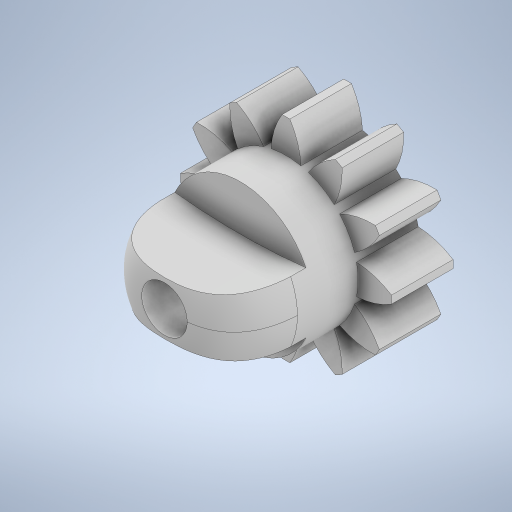
# Autodesk Inventor part: 가스벨브 기어
Saved by Autodesk Inventor 2023.1 (Build 271208000, 208)
## iProperties
Created: 2022-08-14
Part Number: 가스벨브 기어
Material: 일반
Document SubType Name: Modeling
Designer: fly01
Density: 1 g/cm^3
Appearance: 기본값
Author: fly01
Autodesk Inventor part; units mm, degrees
ref_plane "YZ Plane" through (0, 0, 0) normal (1, 0, 0) x (0, 1, 0)
ref_plane "XZ Plane" through (0, 0, 0) normal (0, 1, 0) x (-1, 0, 0)
ref_plane "XY Plane" through (0, 0, 0) normal (0, 0, 1) x (1, 0, 0)
sketch "스케치1" plane through (0, 0, 0) normal (0, 0, 1) x (1, 0, 0)
  circle A0 centre (0, 0) radius 12 construction
  circle A1 centre (0, 0) radius 14
  circle A2 centre (0, 0) radius 9.5
  line L0 (0, 16.0877) -> (0, 8.5475) construction
  line L1 (-0.57, 16.0877) -> (-0.57, 8.5475) construction
  line L2 (-1.57, 16.0877) -> (-1.57, 8.5475) construction
  line L3 (-2.07, 16.0877) -> (-2.07, 8.5475) construction
  arc A3 (-0.57, 13.9884) -> (-2.07, 9.2717) centre (7.6252, 8.7853) ccw
  arc A4 (2.07, 9.2717) -> (0.57, 13.9884) centre (-7.6252, 8.7853) ccw
  circle A5 centre (0, 0) radius 3.75
  line L4 (-3.75, 2.45) -> (3.75, 2.45)
  line L5 (3.75, 2.45) -> (3.75, -2.45)
  line L6 (3.75, -2.45) -> (-3.75, -2.45)
  line L7 (-3.75, -2.45) -> (-3.75, 2.45)
  line L8 (-3.75, 2.45) -> (3.75, -2.45) construction
  line L9 (3.75, 2.45) -> (-3.75, -2.45) construction
  point P0 (2.839, 2.45)
  point P1 (2.839, -2.45)
  point P2 (-2.839, -2.45)
  point P3 (-2.839, 2.45)
  point P4 (2.07, 9.2717)
  point P5 (0.57, 13.9884)
  dimension "d1" = 28
  dimension "d2" = 19
  dimension "d0" = 24
  dimension "d3" = 1.57
  dimension "d4" = 1
  dimension "d5" = 0.5
  dimension "d6" = 7.5
  dimension "d7" = 4.9
  constraints: 20 end point, 5 parallel, 4 centre point, 4 coincident, 4 point on circle, 3 symmetric about line, 2 midpoint, 2 point on line, 1 horizontal, 1 perpendicular, 1 vertical, 1 vertical alignment, 7 other
  measures "d0" diameter of A0
  measures "d3" distance between parallel lines of L0 L2
  measures "d4" distance between parallel lines of L2 L1
  measures "d5" distance between parallel lines of L3 L2
  measures "d6" diameter of A5
  measures "d7" distance of L4.end L5.end
extrude "돌출1" add sketch "스케치1" along normal blind 8.1 contours A2 | A5 L6 L4 | L5 L6 A5 | A5 L4 L5 | L4 A5 | A5 L6 | A5 L7 L4 | L6 L7 A5
extrude "돌출2" add sketch "스케치1" along normal blind 8.1 contours A4 A2 A3 A1 picked at (0.4463, 11.4518)
extrude "돌출3" cut sketch "스케치1" along normal blind 4.1 contours A5 L6 L4
sketch "스케치2" plane through (0, 0, 8.1) normal (0, 0, 1) x (1, 0, 0)
  circle A0 centre (0, 0) radius 1.75
  dimension "d14" = 3.5
  constraints: 1 centre point, 1 coincident
  measures "d14" diameter of A0
extrude "돌출4" cut sketch "스케치2" against normal through all
sketch "스케치4" plane through (0, 0, 8.1) normal (0, 0, 1) x (1, 0, 0)
  circle A0 centre (0, 0) radius 1.75 projected
  arc A1 (-2.07, 9.2717) -> (2.07, 9.2717) centre (0, 0) ccw projected
  arc A2 (2.07, 9.2717) -> (0.57, 13.9884) centre (-7.6252, 8.7853) ccw projected
  arc A3 (0.57, 13.9884) -> (-0.57, 13.9884) centre (0, 0) ccw projected
  arc A4 (-0.57, 13.9884) -> (-2.07, 9.2717) centre (7.6252, 8.7853) ccw projected
  arc A5 (1.9736, 9.1905) -> (0.5135, 13.8905) centre (-7.6252, 8.7853) ccw
  arc A6 (-1.9736, 9.1905) -> (1.9736, 9.1905) centre (0, 0) ccw
  arc A7 (-0.5135, 13.8905) -> (-1.9736, 9.1905) centre (7.6252, 8.7853) ccw
  arc A8 (0.5135, 13.8905) -> (-0.5135, 13.8905) centre (0, 0) ccw
  arc A9 (-0.57, 13.9884) -> (-2.07, 9.2717) centre (7.6252, 8.7853) ccw projected
  circle A10 centre (0, 0) radius 9.5
  point P0 (-1.9687, 9.2938)
  point P1 (1.9687, 9.2938)
  point P2 (2.07, 9.2717)
  dimension "d23" = 0.1
  constraints: 8 point on circle, 4 centre point, 1 coincident, 6 other
  measures "d23" radial gap between concentric circles of A2 A5
extrude "돌출6" cut sketch "스케치4" against normal through all contours A4 A3 A2 A10 A5 A8 A7
pattern_circular "원형 패턴2" count 12 over 360 about axis through (0, 0, 0) along (0, 0, 1) of "돌출6", "돌출2"
sketch "스케치5" plane through (0, 0, 8.1) normal (0, 0, 1) x (1, 0, 0)
  circle A0 centre (0, 0) radius 3
  arc A1 (-1.9687, 9.2938) -> (-2.9419, 9.033) centre (0, 0) ccw projected
  circle A2 centre (0, 0) radius 9.5
  circle A3 centre (0, 0) radius 1.75 projected
  point P0 (-2.9419, 9.033)
  dimension "d29" = 6
  constraints: 2 coincident, 1 centre point, 3 other
  measures "d29" diameter of A0
extrude "돌출7" add sketch "스케치5" along normal blind 16 contours A2 A1
extrude "돌출8" add sketch "스케치5" along normal blind 10 contours A0
sketch "스케치6" plane through (0, 0, 24.1) normal (0, 0, 1) x (1, 0, 0)
  line L0 (0, 0) -> (5.6246, 0)
  arc A0 (7.0643, -6.3519) -> (9.033, -2.9419) centre (0, 0) ccw projected
  arc A1 (-9.033, -2.9419) -> (-7.0643, -6.3519) centre (0, 0) ccw projected
  arc A2 (8.6168, -4) -> (-8.6286, -3.9746) centre (-0.1177, -80.0296) ccw
  circle A3 centre (0, 0) radius 9.5 projected
  arc A4 (-8.6286, 3.9746) -> (8.6168, 4) centre (-0.1177, 80.0296) ccw
  point P0 (-0.0051, -3.5)
  point P1 (-8.6286, 3.9746)
  point P2 (8.6168, 4)
  dimension "d34" = 3.5
  dimension "d35" = 4
  constraints: 7 point on circle, 3 symmetric about line, 2 centre point, 2 end point, 1 horizontal, 1 other
  measures "d34" distance of A3.centre point (-0.005, -3.5)
  measures "d35" vertical distance of L0.start A2.start
extrude "돌출9" cut sketch "스케치6" against normal blind 10 contours A3 A1 A2 A0 | A4 A3
sketch "스케치7" plane through (0, 0, 0) normal (0, 1, 0) x (-1, 0, 0)
  line L0 (-9.5, 8.1) -> (-9.5, 24.1) projected
  spline S0 degree 2 poles (0, 24.1) (-9.0043, 24.9764) (-9.5, 16.1) knots 0 0 0 1 1 1
  line L1 (-9.5, 24.1) -> (0, 24.1)
  line L2 (0, 24.1) -> (0, 28.4108)
  point P0 (0, 0)
  point P1 (-6.9051, 22.5145)
  constraints: 4 end point, 1 horizontal, 1 midpoint, 1 vertical, 3 other
revolve "회전1" cut sketch "스케치7" angle 360 about axis through (0, 0, 24.1) along (0, 0, -1)
